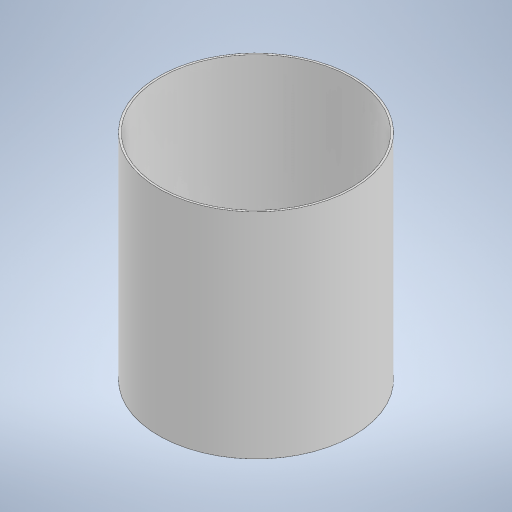
# Autodesk Inventor part: Test_base
Saved by Autodesk Inventor 2024.2 (Build 282272000, 272)
## iProperties
Created: 2024-01-17
Part Number: Test_base
Material: Generic
Document SubType Name: Modeling
Designer: filip
Density: 1 g/cm^3
Appearance: Default
Author: filip
Autodesk Inventor part; units mm, degrees
ref_plane "YZ Plane" through (0, 0, 0) normal (1, 0, 0) x (0, 1, 0)
ref_plane "XZ Plane" through (0, 0, 0) normal (0, 1, 0) x (-1, 0, 0)
ref_plane "XY Plane" through (0, 0, 0) normal (0, 0, 1) x (1, 0, 0)
sketch "Sketch1" plane through (0, 0, 0) normal (0, 1, 0) x (-1, 0, 0)
  circle A0 centre (0, 0) radius 50
  circle A1 centre (0, 0) radius 40
  line L0 (-5, -42.5) -> (5, -42.5)
  line L1 (5, -42.5) -> (5, 42.5)
  line L2 (5, 42.5) -> (-5, 42.5)
  line L3 (-5, 42.5) -> (-5, -42.5)
  line L4 (-5, -42.5) -> (5, 42.5) construction
  line L5 (5, -42.5) -> (-5, 42.5) construction
  line L6 (-42.5, -5) -> (42.5, -5)
  line L7 (42.5, -5) -> (42.5, 5)
  line L8 (42.5, 5) -> (-42.5, 5)
  line L9 (-42.5, 5) -> (-42.5, -5)
  line L10 (-42.5, -5) -> (42.5, 5) construction
  line L11 (42.5, -5) -> (-42.5, 5) construction
  point P0 (5, -5)
  point P1 (39.6863, -5)
  point P2 (5, -39.6863)
  point P3 (-5, 5)
  point P4 (-39.6863, 5)
  point P5 (-5, 39.6863)
  point P6 (-5, -5)
  point P7 (-5, -39.6863)
  point P8 (-39.6863, -5)
  point P9 (5, 5)
  point P10 (5, 39.6863)
  point P11 (39.6863, 5)
  dimension "d0" = 100
  dimension "d1" = 80
  dimension "d2" = 10
  dimension "d3" = 85
  dimension "d4" = 85
  constraints: 24 end point, 4 midpoint, 4 parallel, 2 centre point, 2 coincident, 2 horizontal, 2 perpendicular
  measures "d0" diameter of A0
  measures "d1" diameter of A1
  measures "d2" distance of L2.end L1.end
  measures "d3" distance of L1.end L0.end
  measures "d4" distance of L8.end L7.end
extrude "Extrusion1" add sketch "Sketch1" along normal blind 8 contours A0 | A1 L6 L1 L8 | A1 L8 L7 L6 | L1 L8 L3 A1 | A1 L3 L2 L1 | L1 L6 L3 L8 | L1 L0 L3 A1 | A1 L3 L6 L1 | L3 L6 A1 L8 | A1 L6 L9 L8
sketch "Sketch2" plane through (0, 8, 0) normal (0, 1, 0) x (1, 0, 0)
  point P0 (0, 0)
  point P1 (-8, 0)
  point P2 (0, 0)
  point P3 (0, -8)
  point P4 (8, 0)
  point P5 (0, 8)
  dimension "d7" = 8
  dimension "d40" = 360
  constraints: 1 coincident, 5 other
  measures "d7" distance of point (-8, 0) point (0, 0)
hole "Hole1" at (-8, 8, 0) at (0, 8, -8) at (8, 8, 0) at (0, 8, 8) at (0, 8, 0) direction (0, -1, 0) diameter 5.1 end through all counterbore diameter 6.8 counterbore depth 1
sketch "Sketch6" plane through (0, 0, 0) normal (0, -1, 0) x (1, 0, 0)
  circle A0 centre (0, 8) radius 3.4 projected
  circle A1 centre (8, 0) radius 3.4 projected
  circle A2 centre (0, 0) radius 3.4 projected
  circle A3 centre (-8, 0) radius 3.4 projected
  circle A4 centre (0, -8) radius 3.4 projected
extrude "Extrusion4" cut sketch "Sketch6" against normal blind 1
sketch "Sketch8" plane through (0, 0, 0) normal (0, -1, 0) x (1, 0, 0)
  circle A0 centre (0, 0) radius 50 projected
  circle A1 centre (0, 0) radius 49
  dimension "d45" = 1
  constraints: 1 centre point, 1 coincident
  measures "d45" radial gap between concentric circles of A1 A0
extrude "Extrusion5" add sketch "Sketch8" against normal blind 110
sketch "Sketch5" plane through (0, 0, 0) normal (0, -1, 0) x (1, 0, 0)
  circle A0 centre (0, 0) radius 14.6259
  circle A1 centre (0, 0) radius 68.9057
  constraints: 2 centre point, 2 coincident
body "Solid1"
